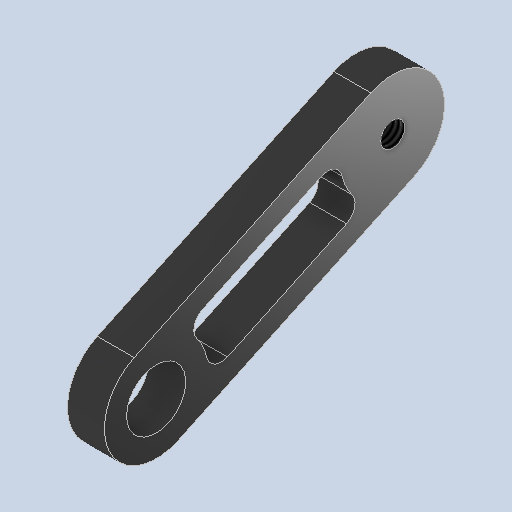
# Autodesk Inventor part: ParallelLinksDriveSimpleFrame
Saved by Autodesk Inventor 2024.2 (Build 282272000, 272)
## iProperties
Created: 2024-04-10
Part Number: ParallelLinksDriveSimpleFrame
Material: Aluminum 7075
Document SubType Name: Modeling
Designer: Masato Kubotera
Density: 2.81 g/cm^3
Appearance: Glossy - Black
Mass: 6.49639 g
Surface Area: 18.8101 cm^2
Volume: 2.31188 cm^3
Vendor: meviy
Author: Masato Kubotera
Autodesk Inventor part; units mm, degrees
ref_plane "YZ Plane" through (0, 0, 0) normal (1, 0, 0) x (0, 1, 0)
ref_plane "XZ Plane" through (0, 0, 0) normal (0, 1, 0) x (-1, 0, 0)
ref_plane "XY Plane" through (0, 0, 0) normal (0, 0, 1) x (1, 0, 0)
derived "ParallelLinksDriveFrame.ipt"
sketch "Sketch1" plane through (0, 0, 0) normal (0, 1, 0) x (-1, 0, 0)
  arc A0 (-2.971, 6.3382) -> (0, -7) centre (0, 0) ccw
  line L0 (0, 0) -> (40, 0) construction
  arc A1 (42.3749, -4.4) -> (42.3749, 4.4) centre (40, 0) ccw
  circle A2 centre (20, 0) radius 20 construction
  circle A3 centre (0, 0) radius 40 construction
  line L1 (42.3749, 4.4) -> (17.6251, 4.4)
  line L2 (0, 0) -> (10, -17.3205) construction
  line L3 (10, -17.3205) -> (20, -34.641) construction
  arc A4 (17.6251, 4.4) -> (17.6251, -4.4) centre (20, 0) ccw
  line L4 (42.3749, -4.4) -> (17.6251, -4.4)
  line L5 (30, 4.4) -> (30, -4.4) construction
  circle A5 centre (40, 0) radius 7 construction
  circle A6 centre (0, 0) radius 7 construction
  circle A7 centre (32, 15) radius 7 construction
  line L6 (-2.971, 6.3382) -> (29.029, 21.3382)
  line L7 (38.1765, 18.2941) -> (46.1765, 3.2941)
  line L8 (0, -7) -> (40, -7)
  arc A8 (40, -7) -> (46.1765, 3.2941) centre (40, 0) ccw
  arc A9 (38.1765, 18.2941) -> (29.029, 21.3382) centre (32, 15) ccw
  arc A10 (43.3651, 3.6981) -> (41.1611, 4.4) centre (41.768, 2.4943) ccw
  arc A11 (41.1611, -4.4) -> (43.3651, -3.6981) centre (41.768, -2.4943) ccw
  arc A12 (18.8389, 4.4) -> (16.6349, 3.6981) centre (18.232, 2.4943) ccw
  arc A13 (16.6349, -3.6981) -> (18.8389, -4.4) centre (18.232, -2.4943) ccw
  circle A14 centre (0, 0) radius 4 construction
sketch "Sketch2" plane through (0, 0, 0) normal (0, 1, 0) x (-1, 0, 0)
  arc A0 (-2.971, 6.3382) -> (2.971, -6.3382) centre (0, 0) ccw
  arc A1 (34.971, 8.6618) -> (29.029, 21.3382) centre (32, 15) ccw
  circle A2 centre (32, 15) radius 7 construction
  circle A3 centre (0, 0) radius 7 construction
  line L0 (-2.971, 6.3382) -> (29.029, 21.3382)
  line L1 (34.971, 8.6618) -> (2.971, -6.3382)
  arc A4 (8.2623, 8.2906) -> (11.6578, 1.0469) centre (9.96, 4.6688) ccw
  arc A5 (23.7377, 6.7094) -> (20.3422, 13.9531) centre (22.04, 10.3312) ccw
  line L2 (3.5037, 6.06) -> (25.1008, 16.1836)
  line L3 (6.8992, -1.1836) -> (28.4963, 8.94)
  line L4 (0, 0) -> (32, 15) construction
  arc A6 (6.8992, -1.1836) -> (3.5037, 6.06) centre (0, 0) ccw
  line L5 (13.029, 13.8382) -> (18.971, 1.1618) construction
  arc A7 (25.1008, 16.1836) -> (28.4963, 8.94) centre (32, 15) ccw
  dimension "d1" = 3
  constraints: 14 point on circle, 12 end point, 10 tangent, 6 centre point, 6 point on line, 3 coincident, 3 symmetric about line, 2 concentric, 2 midpoint, 1 parallel, 2 other
  measures "d1" distance between parallel lines of L2 L0
extrude "Extrusion1" add sketch "Sketch2" along normal blind 5
hole "Hole1" at (-32, 0, 15) direction (0, 1, 0) diameter 3.242 end through all thread size "M4x0.7" class "6H" standard "ANSI Metric M Profile"
fillet "Fillet1" radius 2 4 edges at (-3.5037, 2.5, 6.06) (-6.8992, 2.5, -1.1836) (-25.1008, 2.5, 16.1836) (-28.4963, 2.5, 8.94)
hole "Hole2" at (0, 0, 0) direction (0, 1, 0) diameter 8 end through all
body "Solid1"
